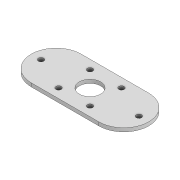
# Autodesk Inventor part: Motor_mount_plate_large
Saved by Autodesk Inventor 2022 (Build 260153000, 153)
## iProperties
Created: 2022-04-28
Part Number: Motor_mount_plate_large
Material: Generic
Document SubType Name: Modeling
Designer: dell
Density: 1 g/cm^3
Appearance: Default
Author: dell
Autodesk Inventor part; units mm, degrees
ref_plane "YZ Plane" through (0, 0, 0) normal (1, 0, 0) x (0, 1, 0)
ref_plane "XZ Plane" through (0, 0, 0) normal (0, 1, 0) x (-1, 0, 0)
ref_plane "XY Plane" through (0, 0, 0) normal (0, 0, 1) x (1, 0, 0)
sketch "Sketch2" plane through (0, 0, 0) normal (0, 1, 0) x (-1, 0, 0)
  line L0 (0, 0) -> (28, 0)
  line L1 (28, 0) -> (28, -28)
  line L2 (28, -28) -> (0, -28)
  line L3 (0, -28) -> (0, 0)
  line L4 (28, 0) -> (0, -28) construction
  line L5 (28, -28) -> (0, 0) construction
  circle A0 centre (22.8388, -5.1612) radius 1.5
  circle A1 centre (22.8388, -22.8388) radius 1.5
  circle A2 centre (5.1612, -5.1612) radius 1.5
  circle A3 centre (5.1612, -22.8388) radius 1.5
  circle A4 centre (14, -14) radius 6
  line L6 (28, -28) -> (33, -28)
  line L7 (33, -28) -> (33, 0)
  line L8 (33, 0) -> (28, 0)
  line L9 (28, 0) -> (28, -28)
  line L10 (0, -28) -> (-5, -28)
  line L11 (-5, -28) -> (-5, 0)
  line L12 (-5, 0) -> (0, 0)
  line L13 (0, 0) -> (0, -28)
  arc A5 (33, -28) -> (33, 0) centre (33, -14) ccw
  arc A6 (-5, 0) -> (-5, -28) centre (-5, -14) ccw
  circle A7 centre (41.5, -14) radius 1.5
  circle A8 centre (-13.5, -14) radius 1.5
  dimension "d37" = 3
  dimension "d38" = 3
  dimension "d39" = 3
  dimension "d40" = 3
  dimension "d41" = 12.5
  dimension "d42" = 12.5
  dimension "d43" = 12.5
  dimension "d44" = 12.5
  dimension "d60" = 28
  dimension "d61" = 12
  dimension "d66" = 5
  dimension "d67" = 5
  dimension "d68" = 3
  dimension "d69" = 3
  dimension "d70" = 8.5
  dimension "d71" = 8.5
  constraints: 28 end point, 9 centre point, 6 parallel, 4 perpendicular, 4 point on circle, 4 point on line, 4 tangent, 3 horizontal, 2 collinear, 1 coincident, 1 midpoint
  measures "d37" diameter of A0
  measures "d38" diameter of A1
  measures "d39" diameter of A2
  measures "d40" diameter of A3
  measures "d41" distance of point (14, -14) A2.centre
  measures "d42" distance of A1.centre point (14, -14)
  measures "d43" distance of A0.centre point (14, -14)
  measures "d44" distance of A3.centre point (14, -14)
  measures "d60" distance of L2.end L0.start
  measures "d61" diameter of A4
  measures "d66" distance of L7.end L8.end
  measures "d67" distance of L11.end L12.end
  measures "d68" diameter of A7
  measures "d69" diameter of A8
  measures "d70" distance of A5.centre A7.centre
  measures "d71" distance of A6.centre A8.centre
extrude "Extrusion2" add sketch "Sketch2" along normal blind 2
sketch "Sketch3" plane through (0, 2, 0) normal (0, 1, 0) x (1, 0, 0)
  line L0 (5, 28) -> (-33, 28) projected
  arc A0 (-33, 28) -> (-33, 0) centre (-33, 14) ccw projected
  line L1 (-33, 0) -> (5, 0) projected
  arc A1 (5, 0) -> (5, 28) centre (5, 14) ccw projected
  circle A2 centre (-22.8388, 22.8388) radius 1.5 projected
  circle A3 centre (-5.1612, 5.1612) radius 1.5 projected
  circle A4 centre (-14, 14) radius 6 projected
  circle A5 centre (-5.1612, 22.8388) radius 1.5 projected
  circle A6 centre (-22.8388, 5.1612) radius 1.5 projected
  circle A7 centre (-41.5, 14) radius 1.5 projected
  circle A8 centre (13.5, 14) radius 1.5 projected
  point P0 (0, 0)
body "Solid2"
